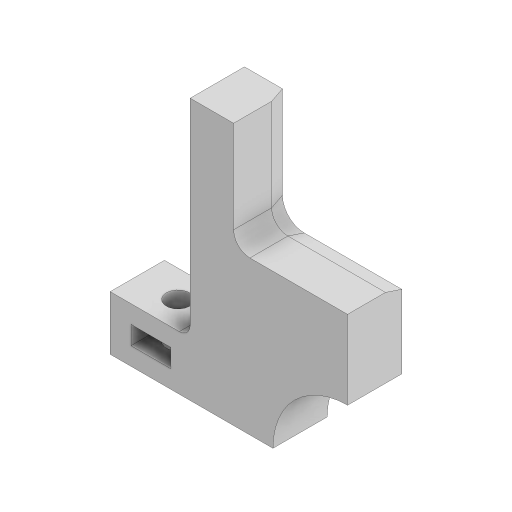
# Autodesk Inventor part: Part2
Saved by Autodesk Inventor 2023.3 (Build 273359000, 359)
## iProperties
Created: 2025-06-02
Part Number: Part2
Material: Generic
Document SubType Name: Modeling
Designer: David Zindović
Density: 1 g/cm^3
Appearance: Default
Author: David Zindović
Autodesk Inventor part; units mm, degrees
ref_plane "YZ Plane" through (0, 0, 0) normal (1, 0, 0) x (0, 1, 0)
ref_plane "XZ Plane" through (0, 0, 0) normal (0, 1, 0) x (-1, 0, 0)
ref_plane "XY Plane" through (0, 0, 0) normal (0, 0, 1) x (1, 0, 0)
sketch "Sketch1" plane through (0, 0, 0) normal (0, 0, 1) x (1, 0, 0)
  arc A0 (0, 13.75) -> (0, -13.75) centre (0, 0) ccw
  line L0 (-18.75, 0) -> (-43.75, 0)
  line L1 (-43.75, 0) -> (-43.75, 10)
  line L2 (-43.75, 10) -> (-18.75, 10)
  line L3 (-18.75, 10) -> (-18.75, 0)
  line L4 (-18.75, 0) -> (-13.75, 0)
  line L5 (-13.75, 0) -> (-13.75, 5)
  line L6 (-13.75, 5) -> (-18.75, 5)
  line L7 (-18.75, 5) -> (-18.75, 0)
  line L8 (-21, 28.25) -> (0, 28.25)
  line L9 (0, 18.75) -> (-21, 18.75)
  line L10 (-21, 18.75) -> (-21, 28.25)
  line L11 (-21, 18.75) -> (-21, 10)
  line L12 (-43.75, 10) -> (-31.25, 10)
  line L13 (-31.25, 0) -> (-43.75, 0)
  line L14 (-43.75, 0) -> (-43.75, 10)
  line L15 (-21, 10) -> (-29, 10)
  line L16 (-29, 10) -> (-29, 48.25)
  line L17 (-29, 48.25) -> (-21, 48.25)
  line L18 (-21, 48.25) -> (-21, 10)
  line L19 (-39.9, 6.7) -> (-32.6, 6.7)
  line L20 (-32.6, 6.7) -> (-32.6, 3.3)
  line L21 (-32.6, 3.3) -> (-39.9, 3.3)
  line L22 (-39.9, 3.3) -> (-39.9, 6.7)
  line L23 (0, -18.75) -> (0, 28.25)
  arc A1 (0, 18.75) -> (0, -18.75) centre (0, 0) ccw
  line L24 (-41.25, 10) -> (-31.25, 10)
  point P0 (-25, 48.25)
  point P1 (-39.9, 5)
  point P2 (-43.75, 5)
  point P3 (-43.75, 5)
  point P4 (-36.25, 6.7)
  dimension "d0" = 27.5
  dimension "d2" = 25
  dimension "d3" = 10
  dimension "d10" = 20
  dimension "d12" = 7.3
  dimension "d13" = 3.4
  dimension "d14" = 8
  dimension "d16" = 5
  dimension "d17" = 5
  dimension "d18" = 21
  dimension "d19" = 5
  dimension "d20" = 21
  dimension "d21" = 9.5
  dimension "d36" = 7.5
  constraints: 50 end point, 10 parallel, 7 horizontal, 6 midpoint, 5 perpendicular, 5 point on circle, 5 point on line, 3 horizontal alignment, 2 centre point, 2 vertical alignment, 1 coincident, 1 tangent, 1 vertical
  measures "d0" diameter of A0
  measures "d2" distance of L1.end L2.end
  measures "d3" distance of L0.end L1.end
  measures "d10" distance from line of point (-25, 48.25) L8
  measures "d12" distance of L20.end L21.end
  measures "d13" distance of L19.end L20.end
  measures "d14" distance of L16.end L17.end
  measures "d16" distance between parallel lines of L4 L6
  measures "d17" distance from line of L3 L5.end
  measures "d18" distance between parallel lines of L18 L23
  measures "d19" radial gap between concentric circles of A1 A0
  measures "d20" distance of L8.start L8.end
  measures "d21" distance between parallel lines of L9 L8
  measures "d36" distance from line of L1 point (-36.25, 6.7)
extrude "Extrusion1" add sketch "Sketch1" along normal blind 10 contours A0 L5 L6 A1 L23 | L4 A1 L6 L5 | A1 L6 L3 L2 L11 L9 | L9 L10 L8 L23 | L0 L1 L2 L3 | L3 L6 A1 | L11 L2 L16 L17 L18 L10
sketch "Sketch2" plane through (-43.75, 0, 0) normal (0, -1, 0) x (1, 0, 0)
  circle A0 centre (7.5, 5) radius 2.15
  line L0 (0, 0) -> (0, 10) projected
  line L1 (0, 0) -> (30, 0) projected
  point P0 (43.75, 0)
  dimension "d26" = 4.3
  dimension "d27" = 7.5
  dimension "d28" = 5
  constraints: 1 centre point
  measures "d26" diameter of A0
  measures "d27" distance from line of L0 A0.centre
  measures "d28" distance from line of L1 A0.centre
extrude "Extrusion2" cut sketch "Sketch2" against normal up to surface (10 mm away)
sketch "Sketch3" plane through (-39.9, 6.7, 0) normal (0, -1, 0) x (1, 0, 0)
  circle A0 centre (3.65, 5) radius 2.15 projected
  line L0 (0, 0) -> (7.3, 0) projected
  line L1 (7.3, 0) -> (7.3, 10) projected
  line L2 (0, 10) -> (7.3, 10) projected
  line L3 (0, 0) -> (0, 10) projected
  line L4 (3.65, 9.0415) -> (7.15, 7.0207)
  line L5 (7.15, 7.0207) -> (7.15, 2.9793)
  line L6 (7.3, 3.0659) -> (3.65, 0.9585)
  line L7 (3.65, 0.9585) -> (0, 3.0659)
  line L8 (0.15, 2.9793) -> (0.15, 7.0207)
  line L9 (0.15, 7.0207) -> (3.65, 9.0415)
  point P0 (39.9, 0)
  point P1 (7, 2.9793)
  point P2 (0, 2.9793)
  dimension "d31" = 7
  dimension "d33" = 0.9586
  constraints: 12 end point, 4 point on line, 1 coincident, 13 other
  measures "d31" distance between parallel lines of L8 L5
  measures "d33" distance from line of L0 L6.end
extrude "Extrusion3" add sketch "Sketch3" along normal up to surface (3.4 mm away) contours L3 L7 L6 L1 L0
fillet "Fillet1" radius 2 1 edges at (-29, 10, 5)
fillet "Fillet2" radius 3 1 edges at (-21, 28.25, 5)
chamfer "Chamfer1" distance 1 distance2 3 3 edges at (-9, 28.25, 0) (-20.1213, 29.1287, 0) (-21, 39.75, 0) measured on face at (-21.5, 39.75, 0) measured on face at (-20.4749, 28.7751, 0) measured on face at (-9, 27.75, 0)
body "Solid1"
